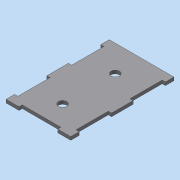
# Autodesk Inventor part: Y-Shafts-Holder_Front-Inner
Saved by Autodesk Inventor 2016 SP1 (Build 200210100, 210)
## iProperties
Created: 2016-01-21
Part Number: Y-Shafts-Holder_Front-Inner
Material: Generic
Document SubType Name: Modeling
Designer: Mohamed A.
Density: 1 g/cm^3
Appearance: Default
Author: Mohamed A.
Autodesk Inventor part; units mm, degrees
ref_plane "YZ Plane" through (0, 0, 0) normal (1, 0, 0) x (0, 1, 0)
ref_plane "XZ Plane" through (0, 0, 0) normal (0, 1, 0) x (-1, 0, 0)
ref_plane "XY Plane" through (0, 0, 0) normal (0, 0, 1) x (1, 0, 0)
sketch "Sketch1" plane through (0, 0, 0) normal (0, 0, 1) x (1, 0, 0)
  circle A0 centre (4.1426, 27.8825) radius 3.9 projected
  circle A1 centre (4.1426, -20.9763) radius 3.9 projected
  line L0 (14.4856, -52.5469) -> (14.4856, -55.5469) construction
  line L1 (14.4856, -55.5469) -> (6.7926, -55.5469) construction
  line L2 (6.7926, -55.5469) -> (6.7926, -52.5469) construction
  line L3 (6.7926, -52.5469) -> (5.6426, -52.5469) projected
  line L4 (5.6426, -52.5469) -> (5.6426, -50.5469) construction
  line L5 (5.6426, -50.5469) -> (6.7926, -50.5469) projected
  line L6 (6.7926, -50.5469) -> (6.7926, -48.1469) projected
  line L7 (6.7926, -48.1469) -> (5.6426, -48.1469) projected
  line L8 (5.6426, -48.1469) -> (5.6426, -47.5469) construction
  line L9 (5.6426, -47.5469) -> (2.6426, -47.5469) construction
  line L10 (2.6426, -47.5469) -> (2.6426, -48.1469) construction
  line L11 (2.6426, -48.1469) -> (1.4926, -48.1469) projected
  line L12 (1.4926, -48.1469) -> (1.4926, -50.5469) projected
  line L13 (1.4926, -50.5469) -> (2.6426, -50.5469) projected
  line L14 (2.6426, -50.5469) -> (2.6426, -52.5469) construction
  line L15 (2.6426, -52.5469) -> (1.4926, -52.5469) projected
  line L16 (1.4926, -52.5469) -> (1.4926, -55.5469) construction
  line L17 (1.4926, -55.5469) -> (-6.2003, -55.5469) construction
  line L18 (-6.2003, -55.5469) -> (-6.2003, -52.5469) construction
  line L19 (-6.2003, -52.5469) -> (-18.7147, -52.5469) construction
  line L20 (-18.7147, -52.5469) -> (-18.7147, -30.9763) construction
  line L21 (-18.7147, -30.9763) -> (-21.7147, -30.9763) construction
  line L22 (-21.7147, -30.9763) -> (-21.7147, -23.6263) construction
  line L23 (-21.7147, -23.6263) -> (-18.7147, -23.6263) construction
  line L24 (-18.7147, -23.6263) -> (-18.7147, -22.4763) projected
  line L25 (-18.7147, -22.4763) -> (-16.7147, -22.4763) construction
  line L26 (-16.7147, -22.4763) -> (-16.7147, -23.6263) projected
  line L27 (-16.7147, -23.6263) -> (-14.3147, -23.6263) projected
  line L28 (-14.3147, -23.6263) -> (-14.3147, -22.4763) projected
  line L29 (-14.3147, -22.4763) -> (-13.7147, -22.4763) construction
  line L30 (-13.7147, -22.4763) -> (-13.7147, -19.4763) construction
  line L31 (-13.7147, -19.4763) -> (-14.3147, -19.4763) construction
  line L32 (-14.3147, -19.4763) -> (-14.3147, -18.3263) projected
  line L33 (-14.3147, -18.3263) -> (-16.7147, -18.3263) projected
  line L34 (-16.7147, -18.3263) -> (-16.7147, -19.4763) projected
  line L35 (-16.7147, -19.4763) -> (-18.7147, -19.4763) construction
  line L36 (-18.7147, -19.4763) -> (-18.7147, -18.3263) projected
  line L37 (-18.7147, -18.3263) -> (-21.7147, -18.3263) construction
  line L38 (-21.7147, -18.3263) -> (-21.7147, -10.9763) construction
  line L39 (-21.7147, -10.9763) -> (-18.7147, -10.9763) construction
  line L40 (-18.7147, -10.9763) -> (-18.7147, 17.8825) construction
  line L41 (-18.7147, 17.8825) -> (-21.7147, 17.8825) construction
  line L42 (-21.7147, 17.8825) -> (-21.7147, 25.2325) construction
  line L43 (-21.7147, 25.2325) -> (-18.7147, 25.2325) construction
  line L44 (-18.7147, 25.2325) -> (-18.7147, 26.3825) projected
  line L45 (-18.7147, 26.3825) -> (-16.7147, 26.3825) construction
  line L46 (-16.7147, 26.3825) -> (-16.7147, 25.2325) projected
  line L47 (-16.7147, 25.2325) -> (-14.3147, 25.2325) projected
  line L48 (-14.3147, 25.2325) -> (-14.3147, 26.3825) projected
  line L49 (-14.3147, 26.3825) -> (-13.7147, 26.3825) construction
  line L50 (-13.7147, 26.3825) -> (-13.7147, 29.3825) construction
  line L51 (-13.7147, 29.3825) -> (-14.3147, 29.3825) construction
  line L52 (-14.3147, 29.3825) -> (-14.3147, 30.5325) projected
  line L53 (-14.3147, 30.5325) -> (-16.7147, 30.5325) projected
  line L54 (-16.7147, 30.5325) -> (-16.7147, 29.3825) projected
  line L55 (-16.7147, 29.3825) -> (-18.7147, 29.3825) construction
  line L56 (-18.7147, 29.3825) -> (-18.7147, 30.5325) projected
  line L57 (-18.7147, 30.5325) -> (-21.7147, 30.5325) construction
  line L58 (-21.7147, 30.5325) -> (-21.7147, 37.8825) construction
  line L59 (-21.7147, 37.8825) -> (-18.7147, 37.8825) construction
  line L60 (-18.7147, 37.8825) -> (-18.7147, 47.8825) projected
  line L61 (-18.7147, 47.8825) -> (27, 47.8825) projected
  line L62 (27, 47.8825) -> (27, 37.8825) projected
  line L63 (27, 37.8825) -> (30, 37.8825) construction
  line L64 (30, 37.8825) -> (30, 30.5325) construction
  line L65 (30, 30.5325) -> (27, 30.5325) construction
  line L66 (27, 30.5325) -> (27, 29.3825) projected
  line L67 (27, 29.3825) -> (25, 29.3825) construction
  line L68 (25, 29.3825) -> (25, 30.5325) projected
  line L69 (25, 30.5325) -> (22.6, 30.5325) projected
  line L70 (22.6, 30.5325) -> (22.6, 29.3825) projected
  line L71 (22.6, 29.3825) -> (22, 29.3825) construction
  line L72 (22, 29.3825) -> (22, 26.3825) construction
  line L73 (22, 26.3825) -> (22.6, 26.3825) construction
  line L74 (22.6, 26.3825) -> (22.6, 25.2325) projected
  line L75 (22.6, 25.2325) -> (25, 25.2325) projected
  line L76 (25, 25.2325) -> (25, 26.3825) projected
  line L77 (25, 26.3825) -> (27, 26.3825) construction
  line L78 (27, 26.3825) -> (27, 25.2325) projected
  line L79 (27, 25.2325) -> (30, 25.2325) construction
  line L80 (30, 25.2325) -> (30, 17.8825) construction
  line L81 (30, 17.8825) -> (27, 17.8825) construction
  line L82 (27, 17.8825) -> (27, -10.9763) construction
  line L83 (27, -10.9763) -> (30, -10.9763) construction
  line L84 (30, -10.9763) -> (30, -18.3263) construction
  line L85 (30, -18.3263) -> (27, -18.3263) construction
  line L86 (27, -18.3263) -> (27, -19.4763) projected
  line L87 (27, -19.4763) -> (25, -19.4763) construction
  line L88 (25, -19.4763) -> (25, -18.3263) projected
  line L89 (25, -18.3263) -> (22.6, -18.3263) projected
  line L90 (22.6, -18.3263) -> (22.6, -19.4763) projected
  line L91 (22.6, -19.4763) -> (22, -19.4763) construction
  line L92 (22, -19.4763) -> (22, -22.4763) construction
  line L93 (22, -22.4763) -> (22.6, -22.4763) construction
  line L94 (22.6, -22.4763) -> (22.6, -23.6263) projected
  line L95 (22.6, -23.6263) -> (25, -23.6263) projected
  line L96 (25, -23.6263) -> (25, -22.4763) projected
  line L97 (25, -22.4763) -> (27, -22.4763) construction
  line L98 (27, -22.4763) -> (27, -23.6263) projected
  line L99 (27, -23.6263) -> (30, -23.6263) construction
  line L100 (30, -23.6263) -> (30, -30.9763) construction
  line L101 (30, -30.9763) -> (27, -30.9763) construction
  line L102 (27, -30.9763) -> (27, -52.5469) construction
  line L103 (27, -52.5469) -> (14.4856, -52.5469) construction
  line L104 (25, 30.5325) -> (22.6, 30.5325)
  line L105 (22.6, 30.5325) -> (22.6, 25.2325)
  line L106 (22.6, 25.2325) -> (25, 25.2325)
  line L107 (25, 25.2325) -> (25, 30.5325)
  line L108 (-14.3147, 30.5325) -> (-16.7147, 30.5325)
  line L109 (-16.7147, 30.5325) -> (-16.7147, 25.2325)
  line L110 (-16.7147, 25.2325) -> (-14.3147, 25.2325)
  line L111 (-14.3147, 25.2325) -> (-14.3147, 30.5325)
  line L112 (-14.3147, -18.3263) -> (-16.7147, -18.3263)
  line L113 (-16.7147, -18.3263) -> (-16.7147, -23.6263)
  line L114 (-16.7147, -23.6263) -> (-14.3147, -23.6263)
  line L115 (-14.3147, -23.6263) -> (-14.3147, -18.3263)
  line L116 (22.6, -18.3263) -> (25, -18.3263)
  line L117 (25, -18.3263) -> (25, -23.6263)
  line L118 (25, -23.6263) -> (22.6, -23.6263)
  line L119 (22.6, -23.6263) -> (22.6, -18.3263)
  line L120 (-21.7147, 14.8825) -> (-18.7147, 14.8825)
  line L121 (-18.7147, -7.9763) -> (-21.7147, -7.9763)
  line L122 (-21.7147, -7.9763) -> (-21.7147, 14.8825)
  line L123 (-18.7147, -33.9763) -> (-21.7147, -33.9763)
  line L124 (-21.7147, -33.9763) -> (-21.7147, -55.5469)
  line L125 (-21.7147, -55.5469) -> (-9.2003, -55.5469)
  line L126 (-9.2003, -55.5469) -> (-9.2003, -52.5469)
  line L127 (17.4856, -52.5469) -> (17.4856, -55.5469)
  line L128 (17.4856, -55.5469) -> (30, -55.5469)
  line L129 (30, -55.5469) -> (30, -33.9763)
  line L130 (30, -33.9763) -> (27, -33.9763)
  line L131 (27, -7.9763) -> (30, -7.9763)
  line L132 (30, -7.9763) -> (30, 14.8825)
  line L133 (30, 14.8825) -> (27, 14.8825)
  line L134 (27, -33.9763) -> (27, -7.9763)
  line L135 (-18.7147, -33.9763) -> (-18.7147, -7.9763)
  line L136 (-9.2003, -52.5469) -> (17.4856, -52.5469)
  line L137 (27, 14.8825) -> (27, 47.8825)
  line L138 (-18.7147, 47.8825) -> (-18.7147, 14.8825)
  line L139 (-18.7147, 47.8825) -> (27, 47.8825)
  line L140 (6.7926, -48.1469) -> (1.4926, -48.1469)
  line L141 (1.4926, -48.1469) -> (1.4926, -50.5469)
  line L142 (1.4926, -50.5469) -> (6.7926, -50.5469)
  line L143 (6.7926, -50.5469) -> (6.7926, -48.1469)
  line L144 (27, 47.8825) -> (30, 47.8825)
  line L145 (30, 47.8825) -> (30, 40.8825)
  line L146 (30, 40.8825) -> (27, 40.8825)
  line L147 (-18.7147, 40.8825) -> (-21.7147, 40.8825)
  line L148 (-21.7147, 40.8825) -> (-21.7147, 47.8825)
  line L149 (-21.7147, 47.8825) -> (-18.7147, 47.8825)
  dimension "d32" = 3
  dimension "d33" = 3
  dimension "d34" = 3
  dimension "d35" = 3
  dimension "d36" = 3
  dimension "d37" = 3
  dimension "d38" = 3
  constraints: 92 end point, 22 point on line, 16 perpendicular, 12 parallel, 8 collinear, 8 horizontal, 1 vertical
  measures "d32" distance between parallel lines of L120 L41
  measures "d33" distance between parallel lines of L39 L121
  measures "d34" distance between parallel lines of L123 L21
  measures "d35" distance between parallel lines of L18 L126
  measures "d36" distance between parallel lines of L0 L127
  measures "d37" distance between parallel lines of L63 L146
  measures "d38" distance between parallel lines of L59 L147
extrude "Extrusion1" add sketch "Sketch1" along normal blind 3
body "Solid1"
